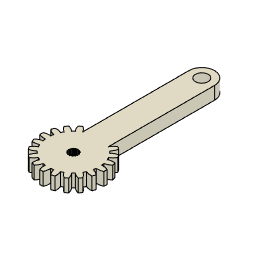
Workshop File v3 (Autodesk Fusion 360 design; units mm, degrees)
Autodesk Fusion 360 part; units mm, degrees
sketch "mount" plane through (0, 0, 0) normal (0, 1, 0) x (1, 0, 0)
  circle A0 centre (0, 0) radius 1.95 construction
  line L0 (0, 0) -> (0, 0.05)
  circle A1 centre (0, 0) radius 12.5
  line L1 (0, 0) -> (0, 12.5) construction
  line L2 (0.3327, 1.565) -> (2.5989, 12.2268)
  line L3 (0, 1.95) -> (0.3327, 1.565)
  line L4 (0, 1.95) -> (-0.3327, 1.565)
  line L5 (-0.3327, 1.565) -> (-2.5989, 12.2268)
  arc A2 (-0.3327, 1.565) -> (0.3327, 1.565) centre (0, 0) ccw construction
  line L6 (0, 0) -> (12.5, 0) construction
  dimension "d1" = 3.9
  dimension "d2" = 3.2
  dimension "d3" = 10.55
  dimension "d4" = 12
  constraint coincident A0.centre L0.start
  constraint concentric A0 A2
  constraint vertical L0
  constraint coincident A1 L1.end
  constraint parallel L0 L1
  constraint coincident A1 L2.end
  constraint coincident A0 L3.start
  constraint coincident L1 L3.start
  constraint symmetric L1 L2.end L5.end
  constraint symmetric L1 L3.start L4.start
  constraint symmetric L1 L2.start L4.end
  constraint coincident A1 L6.end
  constraint perpendicular L0 L6
  measures "d1" diameter of A0
  measures "d2" diameter of A2
  measures "d4" angle of L1 L2
extrude "Extrude1" add sketch "mount" along normal blind 5 contours A1 L2 L3 L4 L5 picked at (0, 8.963) makes body 1
pattern_circular "C-Pattern1" count 15 over 360 about axis through (0, 1.75, 0) along (0, 1, 0) of bodies 1 makes body 2 at (-1.0881, 1.6667, -5.119) makes body 3 at (-6.6608, 0, -5.9974) makes body 4 at (-8.5244, 0, -2.7697) makes body 5 at (-8.9139, 0, 0.9369) makes body 6 at (-7.7622, 0, 4.4815) makes body 7 at (-5.2683, 0, 7.2512) makes body 8 at (-1.8635, 0, 8.7672) makes body 9 at (1.8635, 0, 8.7672) makes body 10 at (5.2683, 0, 7.2512) makes body 11 at (7.7622, 0, 4.4815) makes body 12 at (8.9139, 0, 0.9369) makes body 13 at (8.5244, 0, -2.7697) makes body 14 at (6.6608, 0, -5.9974) makes body 15 at (1.0881, 1.6667, -5.119)
combine "Combine1" operation add target body 1 tool bodies 11 12 2 6 15 4 13 5 7 14 10 8 3 9
fillet "Fillet2" radius 0.1 29 edges at (-0.3327, 2.5, -1.565) (0, 2.5, -1.95) (0.3327, 2.5, -1.565) (0.7931, 2.5, -1.7814) (0.9405, 2.5, -1.2944) (1.4491, 2.5, -1.3048) (1.3856, 2.5, -0.8) (1.8546, 2.5, -0.6026) (1.5912, 2.5, -0.1672) (1.9393, 2.5, 0.2038) (1.5217, 2.5, 0.4944) (1.189, 2.5, 1.0706) (1.1462, 2.5, 1.5776) (0.6508, 2.5, 1.4617) (0.4054, 2.5, 1.9074) (0, 2.5, 1.6) (-0.4054, 2.5, 1.9074) (-0.6508, 2.5, 1.4617) (-1.1462, 2.5, 1.5776) (-1.189, 2.5, 1.0706) (-1.6887, 2.5, 0.975) (-1.5217, 2.5, 0.4944) (-1.9393, 2.5, 0.2038) (-1.5912, 2.5, -0.1672) (-1.8546, 2.5, -0.6026) (-1.3856, 2.5, -0.8) (-1.4491, 2.5, -1.3048) (-0.9405, 2.5, -1.2944) (-0.7931, 2.5, -1.7814) on bodies 1
fillet "Fillet2" radius 0.1 1 edges at (1.6887, 2.5, 0.975) on bodies 1
sketch "teeth" plane through (0, 0, 0) normal (0, 1, 0) x (1, 0, 0)
  circle A0 centre (0, 0) radius 12.5
  circle A1 centre (0, 0) radius 2.5 construction
  line L0 (0, 0) -> (0, 12.5)
  line L1 (0, 0) -> (0.6542, 12.4829) construction
  line L2 (0, 0) -> (0, 0.41)
  line L3 (0, 0) -> (1.3066, 12.4315) construction
  line L4 (0, 0) -> (1.9554, 12.3461)
  circle A2 centre (0, 0) radius 10
  circle A3 centre (0, 0) radius 11.25 construction
  arc A4 (1.0453, 9.9452) -> (0.6542, 12.4829) centre (-3.9658, 10.4719) ccw
  dimension "d45" = 25
  dimension "d46" = 5
  dimension "d47" = 3
  dimension "d48" = 6
  dimension "d49" = 9
  dimension "d50" = 20
  dimension "d51" = 22.5
  constraint coincident A0.centre A1.centre
  constraint concentric A0 A1
  constraint coincident A0 L0.end
  constraint vertical L0
  constraint coincident L0 L2.end
  constraint concentric A1 A3
  constraint coincident A0 L1.end
  constraint coincident A0 L3.end
  constraint coincident A0 L4.end
  constraint tangent L3 A4
  constraint coincident L3 A4.start
  constraint coincident A2 A4.start
  measures "d45" diameter of A0
  measures "d46" diameter of A1
  measures "d47" angle of L0 L1
  measures "d48" angle of L0 L3
  measures "d49" angle of L0 L4
  measures "d50" diameter of A2
  measures "d51" diameter of A3
extrude "Extrude5" add sketch "teeth" along normal blind 5 separate body contours A0 L4 A2 A4 makes body 16
mirror "Mirror2" about plane through (1.5643, 0, -9.8769) normal (0.987688, 0, 0.156434) of bodies 16 merged
pattern_circular "C-Pattern3" count 20 over 360 about axis through (0, 1.75, 0) along (0, 1, 0) of bodies 16 makes body 17 at (-2.0989, 3.3333, -12.3225) makes body 18 at (-5.0177, 3.3333, -11.4487) makes body 19 at (-8.3099, 3.3333, -9.3378) makes body 20 at (-11.2029, 3.3333, -5.5449) makes body 21 at (-12.368, 3.3333, -1.8116) makes body 22 at (-12.3225, 3.3333, 2.0989) makes body 23 at (-11.4487, 3.3333, 5.0177) makes body 24 at (-9.5286, 1.6667, 8.0904) makes body 25 at (-5.0177, 1.6667, 11.4487) makes body 26 at (-2.0989, 1.6667, 12.3225) makes body 27 at (1.8116, 1.6667, 12.368) makes body 28 at (5.0177, 3.3333, 11.4487) makes body 29 at (8.7354, 1.6667, 8.9411) makes body 30 at (11.2029, 3.3333, 5.5449) makes body 31 at (12.3225, 1.6667, 2.0989) makes body 32 at (12.368, 1.6667, -1.8116) makes body 33 at (11.0708, 3.3333, -5.8041) makes body 34 at (9.3378, 3.3333, -8.3099) makes body 35 at (4.7499, 3.3333, -11.5624)
combine "Combine5" operation cut target body 1 tool bodies 16 19 18 17 31 32 30 34 35 33 22 25 27 24 28 20 21 26 29 23
sketch "link" plane through (0, 0, 0) normal (0, 1, 0) x (1, 0, 0)
  line L0 (5, 0) -> (5, 50)
  arc A0 (5, 50) -> (-5, 50) centre (0, 50) ccw
  line L1 (-5, 50) -> (-5, 0)
  arc A1 (-5, 0) -> (5, 0) centre (0, 0) ccw
  line L2 (0, 0) -> (0, 50) construction
  circle A2 centre (0, 50) radius 2.5
  circle A3 centre (0, 0) radius 2.5
  dimension "d39" = 50
  dimension "d40" = 10
  dimension "d41" = 5
  dimension "d42" = 5
  constraint tangent L0 A0
  constraint tangent A0 L1
  constraint parallel L0 L1
  constraint tangent L1 A1
  constraint tangent L0 A1
  constraint vertical L2
  constraint coincident A1.centre L2.start
  constraint concentric A0 A2
  measures "d39" distance of A1.centre A0.centre
  measures "d40" diameter of A0
  measures "d41" diameter of A2
  measures "d42" diameter of A3
extrude "Extrude4" add sketch "link" along normal blind 5 bodies 1
equation "d3 = 5.05 mm + 5.5 mm"
